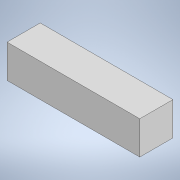
# Autodesk Inventor part: Part5
Saved by Autodesk Inventor 2022 (Build 260153000, 153)
## iProperties
Created: 2022-11-11
Part Number: Part5
Material: Generic
Document SubType Name: Modeling
Designer: trevo
Density: 1 g/cm^3
Appearance: Default
Author: trevo
Autodesk Inventor part; units mm, degrees
ref_plane "YZ Plane" through (0, 0, 0) normal (1, 0, 0) x (0, 1, 0)
ref_plane "XZ Plane" through (0, 0, 0) normal (0, 1, 0) x (-1, 0, 0)
ref_plane "XY Plane" through (0, 0, 0) normal (0, 0, 1) x (1, 0, 0)
sketch "Sketch1" plane through (0, 0, 0) normal (1, 0, 0) x (0, 1, 0)
  line L0 (0, 0) -> (0, 1.27) construction
  line L1 (0, 1.27) -> (1.27, 1.27) construction
  line L2 (0, 0) -> (0, -1.27) construction
  line L3 (0, -1.27) -> (-1.27, -1.27) construction
  line L4 (1.27, 1.27) -> (-1.27, 1.27)
  line L5 (-1.27, 1.27) -> (-1.27, -1.27)
  line L6 (-1.27, -1.27) -> (1.27, -1.27)
  line L7 (1.27, -1.27) -> (1.27, 1.27)
  dimension "d6" = 1.27
  dimension "d7" = 1.27
  dimension "d8" = 1.27
  dimension "d9" = 1.27
  constraints: 16 end point, 3 perpendicular, 2 parallel, 2 vertical, 1 horizontal
  measures "d6" distance of L0.start L0.end
  measures "d7" distance of L0.end L1.end
  measures "d8" distance of L0.start L2.end
  measures "d9" distance of L2.end L3.end
extrude "Extrusion2" add sketch "Sketch1" along normal blind 10.16
body "Solid2"
